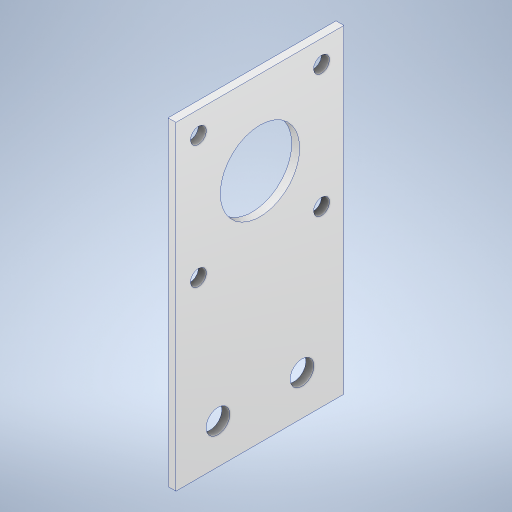
# Autodesk Inventor part: az_rot_mot_holder.iam
Saved by Autodesk Inventor 2024 (Build 280153000, 153)
## iProperties
Created: 2025-12-18
Part Number: az_rot_mot_holder.iam
Material: Aluminum 6061
Document SubType Name: Modeling
Designer: schar
Density: 2.7 g/cm^3
Appearance: Aluminum - Flat
Author: schar
Autodesk Inventor part; units mm, degrees
ref_plane "YZ Plane" through (0, 0, 0) normal (1, 0, 0) x (0, 1, 0)
ref_plane "XZ Plane" through (0, 0, 0) normal (0, 1, 0) x (-1, 0, 0)
ref_plane "XY Plane" through (0, 0, 0) normal (0, 0, 1) x (1, 0, 0)
sketch "Sketch1" plane through (0, 0, 0) normal (1, 0, 0) x (0, 1, 0)
  line L0 (0, 0) -> (-59.252, 0)
  line L1 (-59.252, 0) -> (-59.252, -42.3)
  line L2 (-59.252, -42.3) -> (0, -42.3)
  line L3 (0, -42.3) -> (0, 0)
  line L4 (-59.252, -42.3) -> (-39.252, -42.3)
  line L5 (-39.252, -42.3) -> (-39.252, 0)
  line L6 (-39.252, 0) -> (-59.252, 0)
  line L7 (-59.252, 0) -> (-59.252, -42.3)
  line L8 (-59.252, 0) -> (-49.252, 0)
  line L9 (-49.252, 0) -> (-49.252, -21.15)
  line L10 (-49.252, -21.15) -> (-49.252, -31.725)
  circle A0 centre (-49.252, -31.725) radius 3
  line L11 (-49.252, -21.15) -> (-49.252, -10.575)
  circle A1 centre (-49.252, -10.575) radius 3
  circle A2 centre (0, -21.15) radius 10
  line L12 (0, 0) -> (21.15, 0)
  line L13 (21.15, 0) -> (21.15, -42.3)
  line L14 (21.15, -42.3) -> (0, -42.3)
  line L15 (0, -42.3) -> (0, 0)
  line L16 (0, -21.15) -> (0, -36.65)
  line L17 (0, -36.65) -> (15.5, -36.65)
  circle A3 centre (15.5, -36.65) radius 2
  circle A4 centre (-15.5, -36.65) radius 2
  circle A5 centre (15.5, -5.65) radius 2
  circle A6 centre (-15.5, -5.65) radius 2
  dimension "d1" = 59.252
  dimension "d2" = 42.3
  dimension "d3" = 20
  dimension "d4" = 10
  dimension "d5" = 21.15
  dimension "d6" = 10.575
  dimension "d7" = 6
  dimension "d8" = 10.575
  dimension "d9" = 6
  dimension "d10" = 20
  dimension "d11" = 21.15
  dimension "d12" = 15.5
  dimension "d13" = 15.5
  dimension "d14" = 4
  dimension "d17" = 31
  dimension "d20" = 31
  constraints: 36 end point, 7 centre point, 6 parallel, 5 perpendicular, 4 horizontal, 3 coincident, 3 midpoint, 3 point on line, 1 vertical, 6 other
  measures "d1" distance of L2.end L1.end
  measures "d2" distance of L1.end L0.end
  measures "d3" distance of L6.end L5.end
  measures "d4" distance of L6.end L8.end
  measures "d5" distance of L8.end L9.end
  measures "d6" distance of L9.end L10.end
  measures "d7" diameter of A0
  measures "d8" distance of L9.end L11.end
  measures "d9" diameter of A1
  measures "d10" diameter of A2
  measures "d11" distance of L13.end L14.end
  measures "d12" distance of L16.start L16.end
  measures "d13" distance of L16.end L17.end
  measures "d14" diameter of A3
  measures "d17" distance of A3.centre A4.centre
  measures "d20" distance of A3.centre A5.centre
extrude "Extrusion1" add sketch "Sketch1" along normal blind 2 contours L3 A2 L2 L5 L0 | L12 L13 L14 L3 A2 | L5 L2 L1 L0
body "Solid2"
